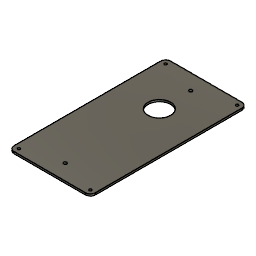
RC car chassis plate (Autodesk Fusion 360 design; units mm, degrees)
part number: 2026-06-28-11-04-36-581
Autodesk Fusion 360 part; units mm, degrees
sketch "Sketch1" plane through (0, 0, 0) normal (0, 0, 1) x (1, 0, 0)
  line L0 (65, 125) -> (-65, 125)
  line L1 (-65, 125) -> (-65, -125)
  line L2 (-65, -125) -> (65, -125)
  line L3 (65, -125) -> (65, 125)
  line L4 (65, 125) -> (-65, -125) construction
  line L5 (-65, 125) -> (65, -125) construction
  dimension "d1" = 130
  dimension "d2" = 250
  constraint horizontal L0
  constraint perpendicular L0 L1
  constraint parallel L0 L2
  constraint parallel L1 L3
  constraint coincident L4 origin
  constraint coincident L5 origin
  measures "d1" distance of L1.end L2.end
  measures "d2" distance of L0.end L1.end
extrude "Extrude1" add sketch "Sketch1" along normal blind 3
sketch "Sketch2" plane through (0, 0, 3) normal (0, 0, 1) x (-1, 0, 0)
  line L0 (-65, 125) -> (-65, -125)
  line L1 (-65, -125) -> (65, -125)
  line L2 (65, -125) -> (65, 125)
  line L3 (65, 125) -> (-65, 125)
  circle A0 centre (0, -50) radius 18
  circle A1 centre (0, -100) radius 2.5
  circle A2 centre (0, 100) radius 2.5
  dimension "d7" = 5
  dimension "d8" = 5
  measures "d7" diameter of A1
  measures "d8" diameter of A2
extrude "Extrude2" cut sketch "Sketch2" against normal blind 3 contours A0 | A1 | A2
fillet "Fillet1" radius 8 4 edges at (65, -125, 1.5) (-65, -125, 1.5) (-65, 125, 1.5) (65, 125, 1.5)
sketch "Sketch3" plane through (0, 0, 3) normal (0, 0, 1) x (-1, 0, 0)
  circle A0 centre (0, 100) radius 2.5
  circle A1 centre (0, -50) radius 18
  circle A2 centre (0, -100) radius 2.5
  arc A3 (-65, -117) -> (-57, -125) centre (-57, -117) ccw
  line L0 (-57, -125) -> (57, -125)
  arc A4 (57, -125) -> (65, -117) centre (57, -117) ccw
  line L1 (65, -117) -> (65, 117)
  arc A5 (65, 117) -> (57, 125) centre (57, 117) ccw
  line L2 (57, 125) -> (-57, 125)
  arc A6 (-57, 125) -> (-65, 117) centre (-57, 117) ccw
  line L3 (-65, 117) -> (-65, -117)
  circle A7 centre (-57, 117) radius 2
  circle A8 centre (57, 117) radius 2
  circle A9 centre (57, -117) radius 2
  circle A10 centre (-57, -117) radius 2
  dimension "d13" = 4
  dimension "d14" = 4
  dimension "d15" = 4
  dimension "d16" = 4
  constraint concentric A6 A7
  constraint concentric A5 A8
  constraint concentric A4 A9
  constraint concentric A3 A10
  measures "d13" diameter of A7
  measures "d14" diameter of A8
  measures "d15" diameter of A9
  measures "d16" diameter of A10
extrude "Extrude3" cut sketch "Sketch3" against normal blind 3 contours A7 | A8 | A9 | A10
